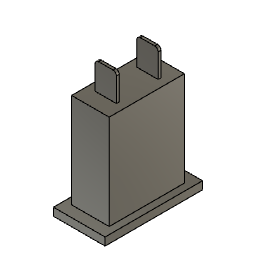
AutomFuseholder (Autodesk Fusion 360 design; units mm, degrees)
Autodesk Fusion 360 part; units mm, degrees
sketch "Sketch1" plane through (0, 0, 0) normal (0, 0, 1) x (1, 0, 0)
  line L0 (7.55, -14.25) -> (-7.55, -14.25)
  line L1 (-7.55, -14.25) -> (-7.55, 14.25)
  line L2 (-7.55, 14.25) -> (7.55, 14.25)
  line L3 (7.55, 14.25) -> (7.55, -14.25)
  line L4 (7.55, -14.25) -> (-7.55, 14.25) construction
  line L5 (-7.55, -14.25) -> (7.55, 14.25) construction
  line L6 (5.5, 11) -> (-5.5, 11)
  line L7 (-5.5, 11) -> (-5.5, -11)
  line L8 (-5.5, -11) -> (5.5, -11)
  line L9 (5.5, -11) -> (5.5, 11)
  line L10 (5.5, 11) -> (-5.5, -11) construction
  line L11 (-5.5, 11) -> (5.5, -11) construction
  line L12 (2.6, -10) -> (-2.6, -10)
  line L13 (-2.6, -10) -> (-2.6, 10)
  line L14 (-2.6, 10) -> (2.6, 10)
  line L15 (2.6, 10) -> (2.6, -10)
  line L16 (2.6, -10) -> (-2.6, 10) construction
  line L17 (-2.6, -10) -> (2.6, 10) construction
  line L18 (5.95, -5.8) -> (-5.95, -5.8)
  line L19 (-5.95, -5.8) -> (-5.95, 5.8)
  line L20 (-5.95, 5.8) -> (5.95, 5.8)
  line L21 (5.95, 5.8) -> (5.95, -5.8)
  line L22 (5.95, -5.8) -> (-5.95, 5.8) construction
  line L23 (-5.95, -5.8) -> (5.95, 5.8) construction
  dimension "d3" = 15.1
  dimension "d4" = 28.5
  dimension "d5" = 11
  dimension "d6" = 22
  dimension "d7" = 5.2
  dimension "d8" = 20
  dimension "d9" = 11.9
  dimension "d10" = 11.6
  constraint horizontal L0
  constraint perpendicular L0 L1
  constraint parallel L0 L2
  constraint parallel L1 L3
  constraint coincident L4 origin
  constraint coincident L5 origin
  constraint horizontal L6
  constraint perpendicular L6 L7
  constraint parallel L6 L8
  constraint parallel L7 L9
  constraint coincident L10 origin
  constraint coincident L11 origin
  constraint horizontal L12
  constraint perpendicular L12 L13
  constraint parallel L12 L14
  constraint parallel L13 L15
  constraint coincident L16 origin
  constraint coincident L17 origin
  constraint horizontal L18
  constraint perpendicular L18 L19
  constraint parallel L18 L20
  constraint parallel L19 L21
  constraint coincident L22 origin
  constraint coincident L23 origin
  measures "d3" distance of L1.end L2.end
  measures "d4" distance of L0.end L1.end
  measures "d5" distance of L7.end L8.end
  measures "d6" distance of L6.end L7.end
  measures "d7" distance of L13.end L14.end
  measures "d8" distance of L12.end L13.end
  measures "d9" distance of L19.end L20.end
  measures "d10" distance of L18.end L19.end
extrude "Extrude2" add sketch "Sketch1" along normal blind 29 contours L6 L7 L9 L13 L14 L15 L20 | L9 L15 L18 L20 | L7 L13 L18 L20 | L7 L8 L9 L12 L13 L15 L18 makes body 1
extrude "Extrude1" add sketch "Sketch1" along normal blind 2.3 contours L0 L1 L2 L3 | L6 L7 L9 L13 L14 L15 L20 | L9 L18 L20 L21 | L7 L18 L19 L20 | L7 L8 L9 L12 L13 L15 L18 bodies 1
sketch "Sketch2" plane through (0, 0, 29) normal (0, 0, 1) x (-1, 0, 0)
  line L0 (2.6, -10) -> (-2.6, -10)
  line L1 (-2.6, -10) -> (-2.6, 10)
  line L2 (-2.6, 10) -> (2.6, 10)
  line L3 (2.6, 10) -> (2.6, -10)
  line L4 (-5.5, 11) -> (-5.5, -11)
  line L5 (-5.5, -11) -> (5.5, -11)
  line L6 (5.5, -11) -> (5.5, 11)
  line L7 (5.5, 11) -> (-5.5, 11)
  line L8 (5.5, -11) -> (-5.5, -11)
  line L9 (-5.5, -11) -> (-5.5, 11)
  line L10 (-5.5, 11) -> (5.5, 11)
  line L11 (5.5, 11) -> (5.5, -11)
  constraint horizontal L8
  constraint vertical L9
  constraint horizontal L10
  constraint vertical L11
  constraint coincident L4.start L7.end
  constraint coincident L5.end L6.start
extrude "Extrude4" add sketch "Sketch2" along normal blind 1 contours L0 L1 L2 L3 | L4 L5 L6 L7 L8 L9 L10 L11 bodies 1
sketch "Sketch3" plane through (0, 0, 30) normal (0, 0, 1) x (-1, 0, 0)
  line L0 (5.5, 11) -> (-5.5, 11)
  line L1 (-5.5, 11) -> (-5.5, -11)
  line L2 (-5.5, -11) -> (5.5, -11)
  line L3 (5.5, -11) -> (5.5, 11)
  line L4 (3.125, -6.5) -> (-3.125, -6.5)
  line L5 (-3.125, -6.5) -> (-3.125, -5.7)
  line L6 (-3.125, -5.7) -> (3.125, -5.7)
  line L7 (3.125, -5.7) -> (3.125, -6.5)
  line L8 (3.125, 5.7) -> (-3.125, 5.7)
  line L9 (-3.125, 5.7) -> (-3.125, 6.5)
  line L10 (-3.125, 6.5) -> (3.125, 6.5)
  line L11 (3.125, 6.5) -> (3.125, 5.7)
  line L12 (-1.75, 0) -> (-22.5, 0)
  line L13 (0, -1.75) -> (0, -22.5)
  dimension "d19" = 0.8
  dimension "d20" = 0.8
  dimension "d21" = 13
  dimension "d22" = 6.25
  dimension "d23" = 6.25
  constraint horizontal L4
  constraint vertical L5
  constraint horizontal L6
  constraint vertical L7
  constraint horizontal L8
  constraint vertical L9
  constraint horizontal L10
  constraint vertical L11
  constraint symmetric L6 L8 L12
  constraint symmetric L5 L7 L13
  constraint symmetric L9 L11 L13
  measures "d19" distance of L4.start L6.end
  measures "d20" distance of L8.start L10.end
  measures "d21" distance of L4 L10
  measures "d22" distance of L5.end L6.end
  measures "d23" distance of L9.end L10.end
extrude "Extrude5" add sketch "Sketch3" along normal blind 8 separate body contours L4 L6 L7 L13 | L4 L5 L6 L13 | L8 L9 L10 L11 makes body 2 at (-1.0417, 6.5, 32.6667) makes body 3 at (-1.0417, -5.7, 32.6667)
fillet "Fillet1" radius 1 4 edges at (3.125, 6.1, 38) (-3.125, 6.1, 38) (-3.125, -6.1, 38) (3.125, -6.1, 38) on bodies 2 3
